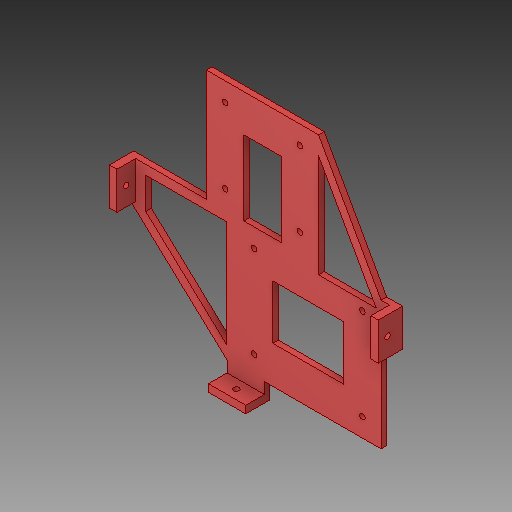
# Autodesk Inventor part: Uchwyt_elektronika
Saved by Autodesk Inventor 2018 (Build 220112000, 112)
## iProperties
Created: 2018-08-20
Part Number: Uchwyt_elektronika
Material: Ogólny
Document SubType Name: Modeling
Designer: Wojciech
Density: 1 g/cm^3
Appearance: Gładki - czerwony
Mass: 28.1305 g
Surface Area: 222.219 cm^2
Volume: 28.1305 cm^3
Author: Wojciech
Autodesk Inventor part; units mm, degrees
ref_plane "YZ Plane" through (0, 0, 0) normal (1, 0, 0) x (0, 1, 0)
ref_plane "XZ Plane" through (0, 0, 0) normal (0, 1, 0) x (-1, 0, 0)
ref_plane "XY Plane" through (0, 0, 0) normal (0, 0, 1) x (1, 0, 0)
sketch "Szkic1" plane through (0, 0, 0) normal (0, 0, 1) x (1, 0, 0)
  line L0 (72, -75) -> (-72, -75)
  line L1 (-72, -75) -> (-72, 75)
  line L2 (-72, 75) -> (72, 75)
  line L3 (72, 75) -> (72, -75)
  line L4 (72, -75) -> (-72, 75) construction
  line L5 (-72, -75) -> (72, 75) construction
  point P0 (0, 0)
  dimension "d0" = 144
  dimension "d1" = 150
  constraints: 12 end point, 2 midpoint, 2 parallel, 1 horizontal, 1 perpendicular
  measures "d0" distance of L1.end L2.end
  measures "d1" distance of L0.end L1.end
extrude "Wyciągnięcie proste1" add sketch "Szkic1" along normal blind 3
sketch "Szkic2" plane through (0, 0, 3) normal (0, 0, 1) x (1, 0, 0)
  line L0 (72, -75) -> (72, 75) projected
  line L1 (-72, -75) -> (72, -75)
  line L2 (72, -75) -> (72, 75)
  line L3 (72, 75) -> (-72, 75)
  line L4 (-72, 75) -> (-72, -75)
  line L5 (-72, -75) -> (72, 75) construction
  line L6 (72, -75) -> (-72, 75) construction
  line L7 (-20, 17.5) -> (20, 17.5)
  line L8 (20, 17.5) -> (20, 57.5)
  line L9 (20, 57.5) -> (-20, 57.5)
  line L10 (-20, 57.5) -> (-20, 17.5)
  point P0 (0, 0)
  point P1 (53.5, -2.5)
  point P2 (53.5, -51.5)
  point P3 (-4.5, -51.5)
  point P4 (-4.5, -2.5)
  dimension "d12" = 58
  dimension "d14" = 58
  dimension "d15" = 49
  dimension "d16" = 18.5
  dimension "d17" = 72.5
  dimension "d18" = 23.5
  dimension "d19" = 18.5
  dimension "d20" = 23.5
  dimension "d21" = 40
  dimension "d22" = 40
  dimension "d23" = 20
  dimension "d24" = 52
  constraints: 20 end point, 4 coincident, 4 parallel, 2 horizontal, 2 midpoint, 2 perpendicular
  measures "d12" distance of point (53.5, -2.5) point (-4.5, -2.5)
  measures "d14" distance of point (53.5, -51.5) point (-4.5, -51.5)
  measures "d15" distance of point (-4.5, -2.5) point (-4.5, -51.5)
  measures "d16" distance from line of L0 point (53.5, -2.5)
  measures "d17" distance from line of L1 point (53.5, -2.5)
  measures "d18" distance from line of L1 point (53.5, -51.5)
  measures "d19" distance from line of L0 point (53.5, -51.5)
  measures "d20" distance from line of L1 point (-4.5, -51.5)
  measures "d21" distance of L9.end L8.end
  measures "d22" distance of L8.end L7.end
  measures "d23" distance from line of point (-4.5, -2.5) L7
  measures "d24" distance between parallel lines of L0 L8
hole "Otwór1" at (53.5, -2.5, 3) at (53.5, -51.5, 3) at (-4.5, -51.5, 3) at (-4.5, -2.5, 3) at (-20, 57.5, 3) at (20, 57.5, 3) at (20, 17.5, 3) at (-20, 17.5, 3) direction (0, 0, -1) diameter 3 end through all
sketch "Szkic3" plane through (0, 0, 3) normal (0, 0, 1) x (1, 0, 0)
  line L0 (-30, 67.5) -> (-10, 67.5)
  line L1 (-10, 75) -> (-10, 7.5)
  line L2 (-10, 7.5) -> (-30, 7.5)
  line L3 (-30, 7.5) -> (-30, 75)
  circle A0 centre (-20, 57.5) radius 1.5 projected
  line L4 (10, 67.5) -> (30, 67.5)
  line L5 (30, 67.5) -> (30, 0)
  line L6 (30, 0) -> (10, 0)
  line L7 (10, 0) -> (10, 67.5)
  circle A1 centre (20, 57.5) radius 1.5 projected
  line L8 (30, 67.5) -> (30, 47.5)
  line L9 (-30, 47.5) -> (-30, 67.5)
  line L10 (-14.5, 7.5) -> (5.5, 7.5)
  line L11 (5.5, 7.5) -> (5.5, -61.5)
  line L12 (5.5, -61.5) -> (-14.5, -61.5)
  line L13 (-14.5, -61.5) -> (-14.5, 7.5)
  circle A2 centre (-4.5, -51.5) radius 1.5 projected
  circle A3 centre (-4.5, -2.5) radius 1.5 projected
  line L14 (-30, 67.5) -> (30, 67.5)
  line L15 (30, 67.5) -> (30, 47.5)
  line L16 (30, 47.5) -> (-30, 47.5)
  line L17 (-30, 47.5) -> (-30, 67.5)
  line L18 (-14.5, 7.5) -> (63.5, 7.5)
  line L19 (63.5, 7.5) -> (63.5, -12.5)
  line L20 (63.5, -12.5) -> (-14.5, -12.5)
  line L21 (-14.5, -12.5) -> (-14.5, 7.5)
  circle A4 centre (53.5, -2.5) radius 1.5 projected
  line L22 (63.5, 7.5) -> (43.5, 7.5)
  line L23 (43.5, 7.5) -> (43.5, -61.5)
  line L24 (43.5, -61.5) -> (63.5, -61.5)
  line L25 (63.5, -61.5) -> (63.5, 7.5)
  circle A5 centre (53.5, -51.5) radius 1.5 projected
  line L26 (-14.5, -61.5) -> (63.5, -61.5)
  line L27 (63.5, -61.5) -> (63.5, -41.5)
  line L28 (63.5, -41.5) -> (-14.5, -41.5)
  line L29 (-14.5, -41.5) -> (-14.5, -61.5)
  line L30 (72, 75) -> (-72, 75) projected
  line L31 (-72, -75) -> (72, -75) projected
  line L32 (-72, 75) -> (72, 75)
  line L33 (72, 75) -> (72, -75)
  line L34 (72, -75) -> (-72, -75)
  line L35 (-72, -75) -> (-72, 75)
  line L36 (-30, 67.5) -> (-10, 67.5)
  line L37 (-10, 67.5) -> (-10, 7.5)
  line L38 (-10, 7.5) -> (-30, 7.5)
  line L39 (-30, 7.5) -> (-30, 67.5)
  point P0 (0, 0)
  dimension "d32" = 20
  dimension "d33" = 10
  dimension "d34" = 20
  dimension "d36" = 10
  dimension "d37" = 20
  dimension "d39" = 20
  dimension "d40" = 10
  dimension "d42" = 10
  dimension "d44" = 10
  dimension "d46" = 10
  dimension "d47" = 10
  dimension "d48" = 60
  dimension "d49" = 20
  dimension "d51" = 78
  dimension "d52" = 10
  dimension "d53" = 20
  dimension "d54" = 20
  dimension "d55" = 78
  dimension "d56" = 20
  constraints: 76 end point, 19 parallel, 9 horizontal, 9 perpendicular, 4 coincident, 3 point on line
  measures "d32" distance of L1.end L2.end
  measures "d33" distance from line of A0.centre L3
  measures "d34" distance of L5.end L6.end
  measures "d36" distance from line of L5 A1.centre
  measures "d37" distance of L8.start L8.end
  measures "d39" distance of L11.end L12.end
  measures "d40" distance from line of L12 A2.centre
  measures "d42" distance from line of L13 A3.centre
  measures "d44" distance from line of L10 A3.centre
  measures "d46" distance from line of A1.centre L4
  measures "d47" distance from line of A0.centre L0
  measures "d48" distance of L8.end L16.end
  measures "d49" distance of L14.end L8.end
  measures "d51" distance of L10.start L18.end
  measures "d52" distance from line of L24 A5.centre
  measures "d53" distance between parallel lines of L25 L23
  measures "d54" distance between parallel lines of L18 L20
  measures "d55" distance of L28.end L27.end
  measures "d56" distance of L27.end L26.end
extrude "Wyciągnięcie proste2" cut sketch "Szkic3" against normal blind 10 contours L3 L30 L1 L0 | L3 L2 L13 L12 L26 L24 L25 L19 L18 L5 L4 L14 L1 L30 L33 L31 L35 | L16 L7 L18 L10 L1 | L20 L23 L28 L11
sketch "Szkic4" plane through (0, 0, 3) normal (0, 0, 1) x (1, 0, 0)
  line L0 (30, 7.5) -> (30, 67.5) projected
  line L1 (63.5, 7.5) -> (63.5, -61.5) projected
  line L2 (30, 67.5) -> (63.5, 7.5)
  line L3 (30, 7.5) -> (63.5, 7.5) projected
  line L4 (63.5, 7.5) -> (30, 7.5)
  line L5 (-30, 67.5) -> (30, 67.5) projected
  line L6 (30, 7.5) -> (30, 67.5)
  line L7 (-19, -71.5) -> (1, -71.5)
  line L8 (1, -71.5) -> (1, -61.5)
  line L9 (1, -61.5) -> (-19, -61.5)
  line L10 (-19, -61.5) -> (-19, -71.5)
  line L11 (-19, -71.5) -> (1, -61.5) construction
  line L12 (1, -71.5) -> (-19, -61.5) construction
  circle A0 centre (-4.5, -51.5) radius 1.5 projected
  line L13 (-19, -61.5) -> (-14.5, -61.5)
  line L14 (-30, 7.5) -> (-30, 67.5) projected
  line L15 (63.5, -12.5) -> (72, -12.5)
  line L16 (72, -12.5) -> (72, 7.5)
  line L17 (72, 7.5) -> (63.5, 7.5)
  line L18 (63.5, 7.5) -> (63.5, -12.5)
  line L19 (63.5, -12.5) -> (72, 7.5) construction
  line L20 (72, -12.5) -> (63.5, 7.5) construction
  circle A1 centre (53.5, -2.5) radius 1.5 projected
  line L21 (-14.5, -61.5) -> (-14.5, 7.5) projected
  line L22 (-14.5, 7.5) -> (-72, 7.5)
  line L23 (-72, 7.5) -> (-72, -12.5)
  line L24 (-72, -12.5) -> (-14.5, -12.5)
  line L25 (-14.5, -12.5) -> (-14.5, 7.5)
  line L26 (-72, -12.5) -> (-19, -61.5)
  line L27 (-14.5, -61.5) -> (-14.5, -12.5)
  point P0 (0, 0)
  point P1 (-9, -66.5)
  point P2 (67.75, -2.5)
  dimension "d59" = 20
  dimension "d60" = 10
  dimension "d61" = 15
  dimension "d62" = 4.5
  dimension "d63" = 8.5
  dimension "d64" = 20
  dimension "d65" = 18.5
  dimension "d67" = 10
  dimension "d68" = 57.5
  dimension "d69" = 20
  constraints: 44 end point, 7 equal length, 5 perpendicular, 4 midpoint, 3 horizontal
  measures "d59" distance of L9.end L8.end
  measures "d60" distance of L8.end L7.end
  measures "d61" vertical distance of A0.centre point (-9, -66.5)
  measures "d62" horizontal distance of A0.centre point (-9, -66.5)
  measures "d63" distance of L17.end L16.end
  measures "d64" distance of L16.end L15.end
  measures "d65" distance from line of A1.centre L16
  measures "d67" distance from line of L3 point (67.75, -2.5)
  measures "d68" distance of L24.end L23.end
  measures "d69" distance of L23.end L22.end
extrude "Wyciągnięcie proste3" add sketch "Szkic4" against normal blind 3 contours L22 L21 L24 L23 | L17 L16 L15 L1 | L0 L2 L3 | L21 L9 L26 L24 | L9 L8 L7 L10
sketch "Szkic5" plane through (0, 0, 3) normal (0, 0, 1) x (1, 0, 0)
  line L0 (63.5, 7.5) -> (72, 7.5) projected
  line L1 (72, 7.5) -> (68, 7.5)
  line L2 (68, 7.5) -> (68, -12.5)
  line L3 (68, -12.5) -> (72, -12.5)
  line L4 (72, -12.5) -> (72, 7.5)
  line L5 (-72, 7.5) -> (-30, 7.5) projected
  line L6 (-72, 7.5) -> (-68, 7.5)
  line L7 (-68, 7.5) -> (-68, -12.5)
  line L8 (-68, -12.5) -> (-72, -12.5)
  line L9 (-72, -12.5) -> (-72, 7.5)
  line L10 (1, -71.5) -> (-19, -71.5) projected
  line L11 (1, -61.5) -> (1, -71.5) projected
  line L12 (-19, -71.5) -> (1, -71.5)
  line L13 (1, -71.5) -> (1, -67.5)
  line L14 (1, -67.5) -> (-19, -67.5)
  line L15 (-19, -67.5) -> (-19, -71.5)
  point P0 (0, 0)
  dimension "d72" = 4
  dimension "d73" = 20
  dimension "d74" = 4
  dimension "d75" = 4
  constraints: 24 end point, 6 parallel, 3 horizontal, 3 perpendicular, 2 point on line
  measures "d72" distance of L3.end L2.end
  measures "d73" distance of L2.end L1.end
  measures "d74" distance of L7.end L8.end
  measures "d75" distance of L13.end L12.end
extrude "Wyciągnięcie proste4" add sketch "Szkic5" along normal blind 10
sketch "Szkic6" plane through (-72, -12.5, 0) normal (-1, 0, 0) x (0, 0, 1)
  line L0 (13, 0) -> (13, 20) projected
  line L1 (0, 20) -> (13, 20) projected
  point P0 (0, 12.5)
  point P1 (8, 10)
  dimension "d78" = 5
  dimension "d79" = 10
  measures "d78" distance from line of L0 point (8, 10)
  measures "d79" distance from line of L1 point (8, 10)
hole "Otwór2" at (-72, -2.5, 8) direction (1, 0, 0) diameter 3 end through all
sketch "Szkic7" plane through (-19, -67.5, 3) normal (0, 1, 0) x (1, 0, 0)
  line L0 (20, -10) -> (0, -10) projected
  line L1 (20, 0) -> (20, -10) projected
  point P0 (19, 3)
  point P1 (10, -5)
  dimension "d87" = 5
  dimension "d88" = 10
  measures "d87" distance from line of L0 point (10, -5)
  measures "d88" distance from line of L1 point (10, -5)
hole "Otwór3" at (-9, -67.5, 8) direction (0, -1, 0) diameter 3 end through all
sketch "Szkic8" plane through (0, 0, 3) normal (0, 0, 1) x (1, 0, 0)
  line L0 (-72, -12.5) -> (-19, -61.5) projected
  line L1 (-19.1082, -54.5905) -> (-19.1082, 2.5)
  line L2 (-19.1082, 2.5) -> (-62.5745, 2.5)
  line L3 (-72, 7.5) -> (-30, 7.5) projected
  line L4 (-62.5745, 2.5) -> (-62.5745, -14.4046)
  line L5 (-62.5745, -14.4046) -> (-19.1082, -54.5905)
  line L6 (-72, 7.5) -> (-72, -12.5) projected
  line L7 (63.5, 7.5) -> (30, 67.5) projected
  line L8 (30, 57.8154) -> (30, 2.5)
  line L9 (30, 57.8154) -> (60.8845, 2.5)
  line L10 (30, 2.5) -> (60.8845, 2.5)
  line L11 (-30, 67.5) -> (-30, 7.5) projected
  point P0 (0, 0)
  dimension "d97" = 5
  dimension "d98" = 16.9046
  dimension "d99" = 40.1859
  dimension "d100" = 9.4254
  dimension "d102" = 5
  dimension "d103" = 55.3154
  dimension "d104" = 60
  constraints: 14 end point, 3 vertical, 2 parallel, 1 horizontal, 1 perpendicular
  measures "d97" distance between parallel lines of L3 L2
  measures "d98" distance of L2.end L4.end
  measures "d99" vertical distance of L4.end L1.start
  measures "d100" distance from line of L6 L4.end
  measures "d102" distance between parallel lines of L3 L10
  measures "d103" vertical distance of L8.start L9.end
  measures "d104" distance between parallel lines of L11 L8
extrude "Wyciągnięcie proste5" cut sketch "Szkic8" against normal blind 10
